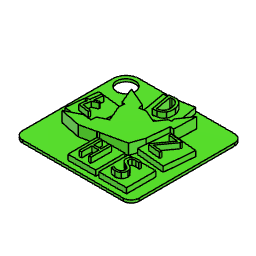
LDZ_Logo v3 (Autodesk Fusion 360 design; units mm, degrees)
Autodesk Fusion 360 part; units mm, degrees
sketch "Sketch1" plane through (0, 0, 0) normal (0, 0, 1) x (1, 0, 0)
  line L0 (-1.3518, 3.8548) -> (1.2546, 4.3161)
  line L1 (1.2546, 4.3161) -> (1.7433, 1.5554)
  line L2 (1.7433, 1.5554) -> (-0.8632, 1.094)
  line L3 (-0.8632, 1.094) -> (-1.3518, 3.8548)
  line L4 (-0.5071, 3.5496) -> (-0.1329, 3.6166)
  spline S0 degree 2 poles (-0.1329, 3.6166) (0.2399, 3.6833) (0.5102, 3.4691) knots 0 0 0 1 1 1
  spline S1 degree 2 poles (0.5102, 3.4691) (0.7802, 3.2563) (0.8595, 2.8135) knots 0 0 0 1 1 1
  spline S2 degree 2 poles (0.8595, 2.8135) (0.9404, 2.3613) (0.7561, 2.0714) knots 0 0 0 1 1 1
  spline S3 degree 2 poles (0.7561, 2.0714) (0.573, 1.783) (0.2164, 1.7192) knots 0 0 0 1 1 1
  line L5 (0.2164, 1.7192) -> (-0.1672, 1.6506)
  line L6 (-0.1672, 1.6506) -> (-0.5071, 3.5496)
  line L7 (0.0191, 1.8825) -> (0.1752, 1.9105)
  spline S4 degree 2 poles (0.1752, 1.9105) (0.4457, 1.9589) (0.5673, 2.1876) knots 0 0 0 1 1 1
  spline S5 degree 2 poles (0.5673, 2.1876) (0.6889, 2.4163) (0.6253, 2.7716) knots 0 0 0 1 1 1
  spline S6 degree 2 poles (0.6253, 2.7716) (0.5622, 3.1243) (0.3672, 3.2977) knots 0 0 0 1 1 1
  spline S7 degree 2 poles (0.3672, 3.2977) (0.1734, 3.4728) (-0.0958, 3.4246) knots 0 0 0 1 1 1
  line L8 (-0.0958, 3.4246) -> (-0.2519, 3.3966)
  line L9 (-0.2519, 3.3966) -> (0.0191, 1.8825)
  line L10 (-4.587, 1.0337) -> (-1.8673, 0.7432)
  line L11 (-1.8673, 0.7432) -> (-2.175, -2.1375)
  line L12 (-2.175, -2.1375) -> (-4.8947, -1.8471)
  line L13 (-4.8947, -1.8471) -> (-4.587, 1.0337)
  line L14 (-2.9712, -1.5752) -> (-4.0118, -1.4347)
  line L15 (-4.0118, -1.4347) -> (-3.9145, -0.7138)
  line L16 (-3.9145, -0.7138) -> (-4.0646, -0.7833)
  line L17 (-4.0646, -0.7833) -> (-4.1424, -0.6238)
  line L18 (-4.1424, -0.6238) -> (-3.886, -0.5025)
  line L19 (-3.886, -0.5025) -> (-3.7537, 0.4772)
  line L20 (-3.7537, 0.4772) -> (-3.5315, 0.4472)
  line L21 (-3.5315, 0.4472) -> (-3.6442, -0.3875)
  line L22 (-3.6442, -0.3875) -> (-3.2346, -0.1944)
  line L23 (-3.2346, -0.1944) -> (-3.1569, -0.3553)
  line L24 (-3.1569, -0.3553) -> (-3.6727, -0.5989)
  line L25 (-3.6727, -0.5989) -> (-3.7634, -1.2709)
  line L26 (-3.7634, -1.2709) -> (-2.945, -1.3814)
  line L27 (-2.945, -1.3814) -> (-2.9712, -1.5752)
  line L28 (-1.0751, -1.7436) -> (-2.7705, 2.2928)
  line L29 (-2.7705, 2.2928) -> (1.444, 0.4491)
  line L30 (1.444, 0.4491) -> (0.6127, -1.4268)
  line L31 (0.6127, -1.4268) -> (-1.0751, -1.7436)
  line L32 (2.1309, 1.0433) -> (4.7842, 0.7982)
  line L33 (4.7842, 0.7982) -> (4.5246, -2.0123)
  line L34 (4.5246, -2.0123) -> (1.8712, -1.7672)
  line L35 (1.8712, -1.7672) -> (2.1309, 1.0433)
  line L36 (3.9135, 0.2126) -> (2.8405, -1.2595)
  line L37 (2.8405, -1.2595) -> (3.7368, -1.3513)
  line L38 (3.7368, -1.3513) -> (3.7169, -1.5458)
  line L39 (3.7169, -1.5458) -> (2.5662, -1.428)
  line L40 (2.5662, -1.428) -> (2.5822, -1.2715)
  line L41 (2.5822, -1.2715) -> (3.6514, 0.2037)
  line L42 (3.6514, 0.2037) -> (2.7823, 0.2927)
  line L43 (2.7823, 0.2927) -> (2.8022, 0.4872)
  line L44 (2.8022, 0.4872) -> (3.9298, 0.3717)
  line L45 (3.9298, 0.3717) -> (3.9135, 0.2126)
  line L46 (-4.2928, -2.7279) -> (0.0305, -0.5881)
  line L47 (0.0305, -0.5881) -> (2.5533, 3.1169)
  line L48 (2.5533, 3.1169) -> (2.4866, 0.534)
  line L49 (2.4866, 0.534) -> (1.5083, -2.2674)
  line L50 (1.5083, -2.2674) -> (-2.367, -3.1205)
  line L51 (-2.367, -3.1205) -> (-4.2928, -2.7279)
  line L52 (-0.9458, -2.759) -> (1.6597, -2.7495)
  line L53 (1.6597, -2.7495) -> (1.6698, -5.5093)
  line L54 (1.6698, -5.5093) -> (-0.9357, -5.5188)
  line L55 (-0.9357, -5.5188) -> (-0.9458, -2.759)
  line L56 (0.8952, -5.1837) -> (0.6709, -5.1824)
  line L57 (0.6709, -5.1824) -> (0.6764, -4.2254)
  line L58 (0.6764, -4.2254) -> (0.016, -4.2216)
  line L59 (0.016, -4.2216) -> (0.0105, -5.1787)
  line L60 (0.0105, -5.1787) -> (-0.2137, -5.1774)
  line L61 (-0.2137, -5.1774) -> (-0.2028, -3.2482)
  line L62 (-0.2028, -3.2482) -> (0.0215, -3.2495)
  line L63 (0.0215, -3.2495) -> (0.0171, -4.0247)
  line L64 (0.0171, -4.0247) -> (0.6775, -4.0285)
  line L65 (0.6775, -4.0285) -> (0.6819, -3.2533)
  line L66 (0.6819, -3.2533) -> (0.9061, -3.2545)
  line L67 (0.9061, -3.2545) -> (0.8952, -5.1837)
  line L68 (1.9525, -2.7352) -> (4.5589, -2.7355)
  line L69 (4.5589, -2.7355) -> (4.5585, -5.4962)
  line L70 (4.5585, -5.4962) -> (1.9521, -5.4959)
  line L71 (1.9521, -5.4959) -> (1.9525, -2.7352)
  spline S8 degree 2 poles (3.6054, -3.3992) (3.4331, -3.3404) (3.2786, -3.3404) knots 0 0 0 1 1 1
  spline S9 degree 2 poles (3.2786, -3.3404) (3.1036, -3.3404) (2.9929, -3.4211) knots 0 0 0 1 1 1
  spline S10 degree 2 poles (2.9929, -3.4211) (2.8835, -3.5004) (2.8835, -3.6481) knots 0 0 0 1 1 1
  spline S11 degree 2 poles (2.8835, -3.6481) (2.8835, -3.8231) (3.172, -3.9557) knots 0 0 0 1 1 1
  spline S12 degree 2 poles (3.172, -3.9557) (3.3853, -4.0542) (3.4537, -4.0924) knots 0 0 0 1 1 1
  spline S13 degree 2 poles (3.4537, -4.0924) (3.5234, -4.1307) (3.5945, -4.1977) knots 0 0 0 1 1 1
  spline S14 degree 2 poles (3.5945, -4.1977) (3.6656, -4.2647) (3.708, -4.3563) knots 0 0 0 1 1 1
  spline S15 degree 2 poles (3.708, -4.3563) (3.7517, -4.4466) (3.7517, -4.56) knots 0 0 0 1 1 1
  spline S16 degree 2 poles (3.7517, -4.56) (3.7517, -4.8417) (3.5617, -4.9976) knots 0 0 0 1 1 1
  spline S17 degree 2 poles (3.5617, -4.9976) (3.373, -5.1521) (3.1159, -5.1521) knots 0 0 0 1 1 1
  spline S18 degree 2 poles (3.1159, -5.1521) (2.8671, -5.1521) (2.6798, -5.0536) knots 0 0 0 1 1 1
  line L72 (2.6798, -5.0536) -> (2.7263, -4.8608)
  spline S19 degree 2 poles (2.7263, -4.8608) (2.9464, -4.9607) (3.1105, -4.9607) knots 0 0 0 1 1 1
  spline S20 degree 2 poles (3.1105, -4.9607) (3.3019, -4.9607) (3.4167, -4.8622) knots 0 0 0 1 1 1
  spline S21 degree 2 poles (3.4167, -4.8622) (3.5329, -4.7624) (3.5329, -4.5888) knots 0 0 0 1 1 1
  spline S22 degree 2 poles (3.5329, -4.5888) (3.5329, -4.4602) (3.4577, -4.3714) knots 0 0 0 1 1 1
  spline S23 degree 2 poles (3.4577, -4.3714) (3.3826, -4.2811) (3.1802, -4.1881) knots 0 0 0 1 1 1
  spline S24 degree 2 poles (3.1802, -4.1881) (2.9724, -4.0924) (2.9108, -4.0583) knots 0 0 0 1 1 1
  spline S25 degree 2 poles (2.9108, -4.0583) (2.8507, -4.0227) (2.7905, -3.9612) knots 0 0 0 1 1 1
  spline S26 degree 2 poles (2.7905, -3.9612) (2.7304, -3.8997) (2.6975, -3.8231) knots 0 0 0 1 1 1
  spline S27 degree 2 poles (2.6975, -3.8231) (2.6647, -3.7465) (2.6647, -3.6563) knots 0 0 0 1 1 1
  spline S28 degree 2 poles (2.6647, -3.6563) (2.6647, -3.417) (2.837, -3.283) knots 0 0 0 1 1 1
  spline S29 degree 2 poles (2.837, -3.283) (3.0093, -3.149) (3.2732, -3.149) knots 0 0 0 1 1 1
  spline S30 degree 2 poles (3.2732, -3.149) (3.466, -3.149) (3.656, -3.2078) knots 0 0 0 1 1 1
  line L73 (3.656, -3.2078) -> (3.6054, -3.3992)
extrude "Extrude1" add sketch "Sketch1" along normal blind 0.5 contours L4 S0 S1 S2 S3 L5 L6 | L14 L15 L16 L17 L18 L19 L20 L21 L22 L23 L24 L25 L26 L27 | L36 L37 L38 L39 L40 L41 L42 L43 L44 L45 | L56 L57 L58 L59 L60 L61 L62 L63 L64 L65 L66 L67 | S8 S9 S10 S11 S12 S13 S14 S15 S16 S17 S18 L72 S19 S20 S21 S22 S23 S24 S25 S26 S27 S28 S29 S30 L73 makes body 1 at (3.2906, -4.0894, 0) makes body 2 at (0.8259, -4.2212, 0) makes body 3 at (2.9386, -0.7798, 0.1667) makes body 4 at (-3.7613, -0.1376, 0) makes body 5 at (-0.3087, 2.8656, 0)
extrude "Extrude2" add sketch "Sketch1" against normal blind 0.5 contours L0 L1 L2 L3 L29 L47 | L2 L3 L29 | L1 L2 L47 | L10 L11 L12 L13 L28 L46 | L10 L11 L28 | L32 L35 L48 L49 | L32 L33 L34 L35 L48 L49 | L11 L12 L46 | L50 L52 L53 L54 L55 | L50 L52 L55 | L68 L69 L70 L71 bodies 1 2 3 4 5
extrude "Extrude3" add sketch "Sketch1" against normal blind 0.5 contours L2 L3 L10 L11 L28 L29 L46 L47 | L1 L2 L11 L12 L28 L29 L30 L31 L32 L35 L46 L47 L48 L49 L50 L51 L52 L55 | L28 L29 L30 L31 L46 L47 bodies 2 3 4 5
extrude "Extrude4" add sketch "Sketch1" along normal blind 0.5 contours L2 L3 L10 L11 L28 L29 L46 L47 | L1 L2 L11 L12 L28 L29 L30 L31 L32 L35 L46 L47 L48 L49 L50 L51 L52 L55 | L28 L29 L30 L31 L46 L47 bodies 2
extrude "Extrude5" add 5 faces at (-3.7613, -0.1376, 0.5) (3.0412, -1.4111, 0.5) (3.2906, -4.0894, 0.5) (0.8259, -4.2212, 0.5) (-0.3087, 2.8656, 0.5) along direction (0, 0, -1) blind 1 on bodies 1 2 bodies 2 1
sketch "Sketch2" plane through (0, 0, -0.5) normal (0, 0, -1) x (1, 0, 0)
  line L0 (-0.2519, -3.3966) -> (0.0191, -1.8825)
  line L1 (0.0191, -1.8825) -> (0.1752, -1.9105)
  spline S0 degree 2 poles (0.1752, -1.9105) (0.4457, -1.9589) (0.5673, -2.1876) knots 0 0 0 1 1 1
  spline S1 degree 2 poles (0.5673, -2.1876) (0.6889, -2.4163) (0.6253, -2.7716) knots 0 0 0 1 1 1
  spline S2 degree 2 poles (0.6253, -2.7716) (0.5622, -3.1243) (0.3672, -3.2977) knots 0 0 0 1 1 1
  spline S3 degree 2 poles (0.3672, -3.2977) (0.1734, -3.4728) (-0.0958, -3.4246) knots 0 0 0 1 1 1
  line L2 (-0.0958, -3.4246) -> (-0.2519, -3.3966)
  line L3 (-1.9185, -0.2643) -> (-2.1234, 1.6542)
  line L4 (-2.1234, 1.6542) -> (-1.2866, 1.24)
  line L5 (-1.2866, 1.24) -> (-1.9185, -0.2643)
  line L6 (1.4553, -1.5044) -> (-0.2701, -1.199)
  line L7 (-0.2701, -1.199) -> (0.8991, -0.6875)
  line L8 (0.8991, -0.6875) -> (1.4553, -1.5044)
  line L9 (-2.1315, -0.7714) -> (-2.7705, -2.2928)
  line L10 (-2.7705, -2.2928) -> (-0.9331, -1.489)
  line L11 (-0.9331, -1.489) -> (-1.3518, -3.8548)
  line L12 (-1.3518, -3.8548) -> (1.2546, -4.3161)
  line L13 (1.2546, -4.3161) -> (1.691, -1.8506)
  line L14 (1.691, -1.8506) -> (2.5533, -3.1169)
  line L15 (2.5533, -3.1169) -> (2.4989, -1.0093)
  line L16 (2.4989, -1.0093) -> (4.7842, -0.7982)
  line L17 (4.7842, -0.7982) -> (4.5246, 2.0123)
  line L18 (4.5246, 2.0123) -> (1.8712, 1.7672)
  line L19 (1.8712, 1.7672) -> (1.939, 1.0341)
  line L20 (1.939, 1.0341) -> (1.5083, 2.2674)
  line L21 (1.5083, 2.2674) -> (-0.7211, 2.7582)
  line L22 (-0.7211, 2.7582) -> (1.6597, 2.7495)
  line L23 (1.6597, 2.7495) -> (1.6698, 5.5093)
  line L24 (1.6698, 5.5093) -> (-0.9357, 5.5188)
  line L25 (-0.9357, 5.5188) -> (-0.9456, 2.8076)
  line L26 (-0.9456, 2.8076) -> (-2.367, 3.1205)
  line L27 (-2.367, 3.1205) -> (-4.2928, 2.7279)
  line L28 (-4.2928, 2.7279) -> (-2.9358, 2.0563)
  line L29 (-2.9358, 2.0563) -> (-4.8947, 1.8471)
  line L30 (-4.8947, 1.8471) -> (-4.587, -1.0337)
  line L31 (-4.587, -1.0337) -> (-2.1315, -0.7714)
  line L32 (-5.5, 6) -> (5.5, 6)
  line L33 (5.5, 6) -> (5.5, -4.5)
  line L34 (5.5, -4.5) -> (-5.5, -4.5)
  line L35 (-5.5, -4.5) -> (-5.5, 6)
  constraint horizontal L32
  constraint vertical L33
  constraint horizontal L34
  constraint vertical L35
extrude "Extrude6" add sketch "Sketch2" along normal blind 0.25 contours L0 L1 S0 S1 S2 S3 L2 | L3 L4 L5 | L6 L7 L8 | L9 L10 L11 L12 L13 L14 L15 L16 L17 L18 L19 L20 L21 L22 L23 L24 L25 L26 L27 L28 L29 L30 L31 | L32 L33 L34 L35 bodies 1 2
hole "Hole1" at (-4.25, 3.25, -0.5) direction (0, 0, -1) diameter 1.75 end through all bodies 1
fillet "Fillet1" radius 0.75 tangency weight 1.00865 2 edges at (5.5, -6, -0.625) (5.5, 4.5, -0.625) on bodies 1
fillet "Fillet2" radius 0.75 1 edges at (-5.5, -6, -0.625) on bodies 1
fillet "Fillet3" radius 1.25 1 edges at (-5.5, 4.5, -0.625) on bodies 1
